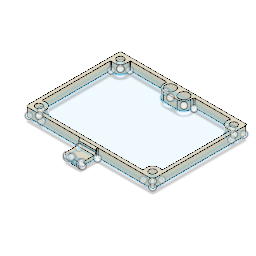
iot-data-logger-enclosure-gasket v4 (Autodesk Fusion 360 design; units mm, degrees)
Autodesk Fusion 360 part; units mm, degrees
sketch "Sketch1" plane through (0, 0, 0) normal (0, 1, 0) x (1, 0, 0)
  line L0 (1, 0) -> (74, 0)
  line L1 (75, -1) -> (75, -55)
  line L2 (0, -55) -> (0, -1)
  circle A0 centre (4, -4) radius 2
  line L3 (2, -48) -> (2, -8)
  arc A1 (7.7004, -53.519) -> (2.481, -48.2996) centre (4, -52) ccw
  arc A2 (0, -51.9989) -> (0, -52.0011) centre (4, -52) ccw
  arc A3 (0, -55) -> (1, -56) centre (1, -55) ccw
  arc A4 (2.481, -48.2996) -> (2, -48) centre (2, -48.5359) ccw
  arc A5 (8, -54) -> (7.7004, -53.519) centre (7.4641, -54) ccw
  circle A6 centre (4, -52) radius 2
  circle A7 centre (71, -52) radius 2
  line L4 (67, -54) -> (8, -54)
  line L5 (73, -8) -> (73, -48)
  arc A8 (72.519, -48.2996) -> (67.2996, -53.519) centre (71, -52) ccw
  arc A9 (74, -56) -> (75, -55) centre (74, -55) ccw
  arc A10 (73, -48) -> (72.519, -48.2996) centre (73, -48.5359) ccw
  arc A11 (67.2996, -53.519) -> (67, -54) centre (67.5359, -54) ccw
  circle A12 centre (71, -4) radius 2
  arc A13 (75, -1) -> (74, 0) centre (74, -1) ccw
  arc A14 (67.2996, -2.481) -> (72.519, -7.7004) centre (71, -4) ccw
  arc A15 (67, -2) -> (67.2996, -2.481) centre (67.5359, -2) ccw
  arc A16 (72.519, -7.7004) -> (73, -8) centre (73, -7.4641) ccw
  arc A17 (2.481, -7.7004) -> (7.7004, -2.481) centre (4, -4) ccw
  arc A18 (2.481, -7.7004) -> (7.7004, -2.481) centre (4, -4) ccw
  arc A19 (1, 0) -> (0, -1) centre (1, -1) ccw
  arc A20 (2, -8) -> (2.481, -7.7004) centre (2, -7.4641) ccw
  arc A21 (7.7004, -2.481) -> (8, -2) centre (7.4641, -2) ccw
  line L6 (45.5, -2.4997) -> (45.5, -4)
  line L7 (29.5, -2.5) -> (29.5, -4)
  arc A22 (29.5, -2.5) -> (29, -2) centre (29, -2.5) ccw
  arc A23 (46, -2) -> (45.5, -2.5003) centre (46, -2.5) ccw
  line L8 (29, -2) -> (8, -2)
  line L9 (67, -2) -> (46, -2)
  arc A24 (29.5, -4) -> (33.5, -8) centre (33.5, -4) ccw
  arc A25 (41.5, -8) -> (45.5, -4) centre (41.5, -4) ccw
  arc A26 (41.5015, 0) -> (41.4985, 0) centre (41.5, -4) ccw
  line L10 (33.5, -8) -> (41.5, -8)
  circle A27 centre (33.5, -4) radius 3
  circle A28 centre (41.5, -4) radius 3
  line L11 (32.5, -56.5) -> (32.5, -65)
  line L12 (33.5, -66) -> (41.5, -66)
  line L13 (42.5, -65) -> (42.5, -56.5)
  line L14 (33.5, -66) -> (41.5, -66)
  line L15 (74, -56) -> (43, -56)
  line L16 (32, -56) -> (1, -56)
  arc A29 (32.5, -56.5) -> (32, -56) centre (32, -56.5) ccw
  arc A30 (43, -56) -> (42.5, -56.5) centre (43, -56.5) ccw
  arc A31 (32.5, -65) -> (33.5, -66) centre (33.5, -65) ccw
  arc A32 (41.5, -66) -> (42.5, -65) centre (41.5, -65) ccw
  line L17 (42.5, -65) -> (42.5, -64.0151)
  line L18 (32.5, -64.0151) -> (32.5, -65)
  line L19 (35, -64) -> (40, -64)
  line L20 (40, -63) -> (35, -63)
  line L21 (34.5, -62) -> (40.5, -62)
  line L22 (41.5, -63) -> (41.5, -64)
  line L23 (40.5, -65) -> (34.5, -65)
  line L24 (33.5, -64) -> (33.5, -63)
  arc A33 (34.5, -62) -> (33.5, -63) centre (34.5, -63) ccw
  arc A34 (40.5, -65) -> (41.5, -64) centre (40.5, -64) ccw
  arc A35 (40, -64) -> (40, -63) centre (40, -63.5) ccw
  arc A36 (41.5, -63) -> (40.5, -62) centre (40.5, -63) ccw
  arc A37 (33.5, -64) -> (34.5, -65) centre (34.5, -64) ccw
  arc A38 (35, -63) -> (35, -64) centre (35, -63.5) ccw
  line L25 (32.5, -57) -> (42.5, -57)
  dimension "d2" = 4
  dimension "d3" = 4
  dimension "d20" = 6
  dimension "d21" = 6
  constraint horizontal L0
  constraint vertical L1
  constraint horizontal L15
  constraint vertical L2
  constraint tangent L2 A18
  constraint concentric A0 A17
  constraint coincident L2 A2.start
  constraint concentric A1 A2
  constraint coincident L2 A2.end
  constraint tangent L2 A3
  constraint concentric A2 A6
  constraint concentric A7 A8
  constraint perpendicular L5 L15
  constraint tangent A9 L15
  constraint perpendicular L2 L9
  constraint tangent L0 A13
  constraint concentric A12 A14
  constraint tangent L0 A14
  constraint tangent L0 A19
  constraint tangent A24 A25
  constraint tangent L6 A25
  constraint tangent L7 A24
  constraint tangent A22 L9
  constraint tangent A23 L9
  constraint coincident A22.end L9
  constraint coincident L6 A23.end
  constraint collinear L8 L9
  constraint coincident A23 L6.start
  constraint coincident L0 A26.end
  constraint coincident L0 A26.start
  constraint concentric A25 A26
  constraint tangent A25 L10
  constraint concentric A24 A27
  constraint concentric A25 A28
  constraint vertical L11
  constraint horizontal L12
  constraint vertical L13
  constraint horizontal L14
  constraint collinear L15 L16
  constraint tangent L16 A29
  constraint tangent L15 A30
  constraint tangent L11 A31
  constraint tangent L13 A32
  constraint vertical L17
  constraint vertical L18
  constraint coincident L13 L17.end
  constraint horizontal L19
  constraint horizontal L20
  constraint horizontal L21
  constraint vertical L22
  constraint horizontal L23
  constraint vertical L24
  constraint tangent L21 A33
  constraint tangent L23 A37
  constraint tangent L23 A34
  constraint coincident L11 L25.start
  constraint coincident L13 L25.end
  constraint perpendicular L13 L25
  measures "d2" diameter of A6 A9.start
  measures "d3" diameter of A7
  measures "d20" diameter of A27
  measures "d21" diameter of A28
extrude "Extrude2" add sketch "Sketch1" along normal blind 2 and the other way blind 0 contours L21 L22 L23 L24 A33 A34 A36 A37 makes body 1
extrude "Extrude3" add sketch "Sketch1" along normal blind 2 contours L11 L12 L13 L14 A31 A32 L17 L18 L25 bodies 1
extrude "Extrude4" add sketch "Sketch1" along normal blind 5 contours L0 L1 L2 A2 A3 A9 A13 A19 A26 L11 L13 L15 L16 A29 A30 L25 bodies 1
extrude "Extrude5" add sketch "Sketch1" along normal blind 2 and the other way blind 3 separate body contours L19 L20 A35 A38 makes body 2
fillet "Fillet1" radius 1 1 edges at (37.5, 2, 57) on bodies 1
combine "Combine1" operation add target body 1 tool bodies 2
fillet "Fillet2" radius 1 1 edges at (37.5, 5, 57) on bodies 1
named bodies: "gasket-tpu"
